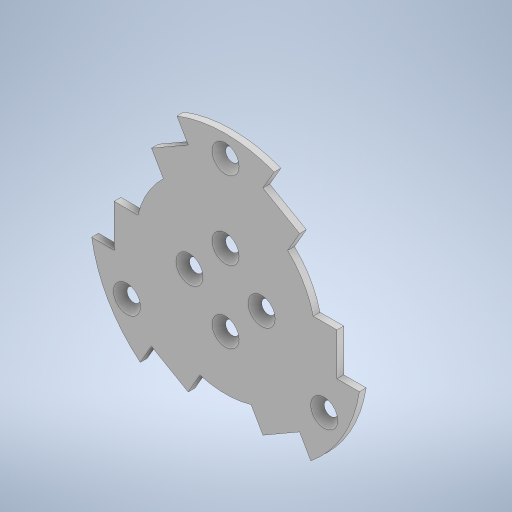
# Autodesk Inventor part: top_part_wheel
Saved by Autodesk Inventor 2023 (Build 270158000, 158)
## iProperties
Created: 2026-02-22
Part Number: top_part_wheel
Material: Типовые
Document SubType Name: Modeling
Designer: garin
Density: 1 g/cm^3
Appearance: По умолчанию
Author: garin
Autodesk Inventor part; units mm, degrees
ref_plane "YZ Plane" through (0, 0, 0) normal (1, 0, 0) x (0, 1, 0)
sketch "Эскиз1" plane through (0, 0, 0) normal (0, 0, 1) x (1, 0, 0)
  circle A0 centre (0, 0) radius 35
  circle A1 centre (0, 0) radius 20
  line L0 (0, 0) -> (34.5691, 5.4752) construction
  line L1 (0, 0) -> (35, 0) construction
  line L2 (0, 0) -> (34.5691, -5.4752) construction
  line L3 (34.5691, 5.4752) -> (29.6307, 4.693) construction
  line L4 (29.6307, 4.693) -> (19.4416, 4.693)
  line L5 (19.4416, 4.693) -> (34.6839, 4.693)
  line L6 (19.4416, -4.693) -> (34.6839, -4.693)
  line L7 (13.7851, 14.4904) -> (21.4063, 27.6907) construction
  line L8 (10.751, 28.0074) -> (5.6565, 19.1834) construction
  line L9 (5.6565, 19.1834) -> (13.2777, 32.3837) construction
  line L10 (-5.6565, 19.1834) -> (-13.2777, 32.3837) construction
  line L11 (-18.8796, 23.3144) -> (-13.7851, 14.4904) construction
  line L12 (-13.7851, 14.4904) -> (-21.4063, 27.6907) construction
  line L13 (-19.4416, 4.693) -> (-34.6839, 4.693) construction
  line L14 (-29.6307, -4.693) -> (-19.4416, -4.693) construction
  line L15 (-19.4416, -4.693) -> (-34.6839, -4.693) construction
  line L16 (-13.7851, -14.4904) -> (-21.4063, -27.6907) construction
  line L17 (-10.751, -28.0074) -> (-5.6565, -19.1834) construction
  line L18 (-5.6565, -19.1834) -> (-13.2777, -32.3837) construction
  line L19 (5.6565, -19.1834) -> (13.2777, -32.3837) construction
  line L20 (18.8796, -23.3144) -> (13.7851, -14.4904) construction
  line L21 (13.7851, -14.4904) -> (21.4063, -27.6907) construction
  line L22 (0, 0) -> (17.5, 30.3109) construction
  line L23 (0, 0) -> (-17.5, 30.3109) construction
  line L24 (0, 0) -> (-35, 0) construction
  line L25 (0, 0) -> (-17.5, -30.3109) construction
  line L26 (0, 0) -> (17.5, -30.3109) construction
  line L27 (34.6839, 4.693) -> (29.6839, 4.693) construction
  line L28 (29.6839, 4.693) -> (29.6839, -4.693)
  line L29 (29.6839, 4.693) -> (29.6839, 1.693)
  line L30 (29.6839, 1.693) -> (34.959, 1.693)
  line L31 (29.6839, -4.693) -> (29.6839, -1.693) construction
  line L32 (29.6839, -1.693) -> (34.959, -1.693)
  line L33 (13.7851, 14.4904) -> (21.4063, 27.6907)
  line L34 (10.751, 28.0074) -> (5.6565, 19.1834)
  line L35 (13.3758, 26.5536) -> (16.0133, 31.1219)
  line L36 (5.6565, 19.1834) -> (13.2777, 32.3837)
  line L37 (10.7777, 28.0536) -> (18.9063, 23.3605)
  line L38 (16.3082, 24.8605) -> (18.9457, 29.4289)
  line L39 (-5.6565, 19.1834) -> (-13.2777, 32.3837)
  line L40 (-18.8796, 23.3144) -> (-13.7851, 14.4904)
  line L41 (-16.3082, 24.8605) -> (-18.9457, 29.4289)
  line L42 (-13.7851, 14.4904) -> (-21.4063, 27.6907)
  line L43 (-18.9063, 23.3605) -> (-10.7777, 28.0536)
  line L44 (-13.3758, 26.5536) -> (-16.0133, 31.1219)
  line L45 (-19.4416, 4.693) -> (-34.6839, 4.693)
  line L46 (-29.6307, -4.693) -> (-19.4416, -4.693)
  line L47 (-29.6839, -1.693) -> (-34.959, -1.693)
  line L48 (-19.4416, -4.693) -> (-34.6839, -4.693)
  line L49 (-29.6839, -4.693) -> (-29.6839, 4.693)
  line L50 (-29.6839, 1.693) -> (-34.959, 1.693)
  line L51 (-13.7851, -14.4904) -> (-21.4063, -27.6907)
  line L52 (-10.751, -28.0074) -> (-5.6565, -19.1834)
  line L53 (-13.3758, -26.5536) -> (-16.0133, -31.1219)
  line L54 (-5.6565, -19.1834) -> (-13.2777, -32.3837)
  line L55 (-10.7777, -28.0536) -> (-18.9063, -23.3605)
  line L56 (-16.3082, -24.8605) -> (-18.9457, -29.4289)
  line L57 (5.6565, -19.1834) -> (13.2777, -32.3837)
  line L58 (18.8796, -23.3144) -> (13.7851, -14.4904)
  line L59 (16.3082, -24.8605) -> (18.9457, -29.4289)
  line L60 (13.7851, -14.4904) -> (21.4063, -27.6907)
  line L61 (18.9063, -23.3605) -> (10.7777, -28.0536)
  line L62 (13.3758, -26.5536) -> (16.0133, -31.1219)
  circle A2 centre (0, 0) radius 30.0525
  line L63 (21.4063, 27.6907) -> (19.9136, 25.1053) construction
  line L64 (18.9457, 29.4289) -> (17.4457, 26.8308) construction
  line L65 (17.4457, 26.8308) -> (21.2118, 27.8399)
  line L66 (0, 0) -> (21.2118, 27.8399) construction
  line L67 (21.2384, 23.9411) -> (21.2118, 27.8399)
  line L68 (24.7499, 20.2901) -> (25.3388, 24.1443)
  line L69 (21.4607, 23.742) -> (25.3388, 24.1443)
  line L70 (27.6414, 16.1308) -> (28.831, 19.8437)
  line L71 (24.938, 20.0584) -> (28.831, 19.8437)
  line L72 (29.8403, 11.5673) -> (31.6009, 15.046)
  line L73 (27.7906, 15.8723) -> (31.6009, 15.046)
  line L74 (31.2917, 6.714) -> (33.5791, 9.8714)
  line L75 (29.9469, 11.2885) -> (33.5791, 9.8714)
  line L76 (31.9591, 1.6925) -> (34.716, 4.4494)
  line L77 (31.3529, 6.4219) -> (34.716, 4.4494)
  circle A3 centre (0, 0) radius 32.0038
  line L78 (-14.5133, 28.5238) -> (-13.5042, 32.2899)
  line L79 (-10.1144, 30.3635) -> (-13.5042, 32.2899)
  line L80 (-9.8308, 30.4565) -> (-8.2401, 34.0162)
  line L81 (-5.1968, 31.5791) -> (-8.2401, 34.0162)
  line L82 (14.5138, 28.5236) -> (13.5047, 32.2897)
  line L83 (10.1149, 30.3634) -> (13.5047, 32.2897)
  line L84 (9.8313, 30.4564) -> (8.2407, 34.016)
  line L85 (5.1973, 31.579) -> (8.2407, 34.016)
  line L86 (4.9026, 31.6261) -> (2.7702, 34.8902)
  line L87 (0.1495, 32.0035) -> (2.7702, 34.8902)
  line L88 (-0.149, 32.0035) -> (-2.7697, 34.8902)
  line L89 (-4.9021, 31.6262) -> (-2.7697, 34.8902)
  line L90 (-31.959, 1.693) -> (-34.716, 4.45)
  line L91 (-31.3528, 6.4224) -> (-34.716, 4.45)
  line L92 (-31.2916, 6.7145) -> (-33.5789, 9.8719)
  line L93 (-29.9467, 11.289) -> (-33.5789, 9.8719)
  line L94 (-17.4453, 26.8311) -> (-21.2113, 27.8403)
  line L95 (-21.238, 23.9415) -> (-21.2113, 27.8403)
  line L96 (-21.4603, 23.7424) -> (-25.3384, 24.1447)
  line L97 (-24.7496, 20.2905) -> (-25.3384, 24.1447)
  line L98 (-24.9377, 20.0588) -> (-28.8307, 19.8442)
  line L99 (-27.6411, 16.1312) -> (-28.8307, 19.8442)
  line L100 (-27.7903, 15.8727) -> (-31.6007, 15.0465)
  line L101 (-29.8401, 11.5678) -> (-31.6007, 15.0465)
  line L102 (-17.4457, -26.8308) -> (-21.2118, -27.8399)
  line L103 (-21.2384, -23.9411) -> (-21.2118, -27.8399)
  line L104 (-21.4607, -23.742) -> (-25.3388, -24.1443)
  line L105 (-24.7499, -20.2901) -> (-25.3388, -24.1443)
  line L106 (-31.9591, -1.6925) -> (-34.716, -4.4494)
  line L107 (-31.3529, -6.4219) -> (-34.716, -4.4494)
  line L108 (-31.2917, -6.714) -> (-33.5791, -9.8714)
  line L109 (-29.9469, -11.2885) -> (-33.5791, -9.8714)
  line L110 (-29.8403, -11.5673) -> (-31.6009, -15.046)
  line L111 (-27.7906, -15.8723) -> (-31.6009, -15.046)
  line L112 (-27.6414, -16.1308) -> (-28.831, -19.8437)
  line L113 (-24.938, -20.0584) -> (-28.831, -19.8437)
  line L114 (14.5133, -28.5238) -> (13.5042, -32.2899)
  line L115 (10.1144, -30.3635) -> (13.5042, -32.2899)
  line L116 (9.8308, -30.4565) -> (8.2401, -34.0162)
  line L117 (5.1968, -31.5791) -> (8.2401, -34.0162)
  line L118 (-14.5138, -28.5236) -> (-13.5047, -32.2897)
  line L119 (-10.1149, -30.3634) -> (-13.5047, -32.2897)
  line L120 (-9.8313, -30.4564) -> (-8.2407, -34.016)
  line L121 (-5.1973, -31.579) -> (-8.2407, -34.016)
  line L122 (-4.9026, -31.6261) -> (-2.7702, -34.8902)
  line L123 (-0.1495, -32.0035) -> (-2.7702, -34.8902)
  line L124 (0.149, -32.0035) -> (2.7697, -34.8902)
  line L125 (4.9021, -31.6262) -> (2.7697, -34.8902)
  line L126 (31.959, -1.693) -> (34.716, -4.45)
  line L127 (31.3528, -6.4224) -> (34.716, -4.45)
  line L128 (31.2916, -6.7145) -> (33.5789, -9.8719)
  line L129 (29.9467, -11.289) -> (33.5789, -9.8719)
  line L130 (17.4453, -26.8311) -> (21.2113, -27.8403)
  line L131 (21.238, -23.9415) -> (21.2113, -27.8403)
  line L132 (21.4603, -23.7424) -> (25.3384, -24.1447)
  line L133 (24.7496, -20.2905) -> (25.3384, -24.1447)
  line L134 (24.9377, -20.0588) -> (28.8307, -19.8442)
  line L135 (27.6411, -16.1312) -> (28.8307, -19.8442)
  line L136 (27.7903, -15.8727) -> (31.6007, -15.0465)
  line L137 (29.8401, -11.5678) -> (31.6007, -15.0465)
  circle A4 centre (0, 0) radius 11 construction
  line L138 (0, 0) -> (0, 8) construction
  circle A5 centre (0, 8) radius 1.5
  circle A6 centre (0, -8) radius 1.5
  line L139 (0, 0) -> (8, 0) construction
  circle A7 centre (8, 0) radius 1.5
  circle A8 centre (-8, 0) radius 1.5
  circle A9 centre (0, 0) radius 12.5
  line L140 (-10.751, -28.0074) -> (-9.251, -25.4093)
  circle A10 centre (0, 0) radius 27.041
  line L141 (24.7024, 4.693) -> (24.7024, -4.693)
  line L142 (8.2869, 23.7395) -> (16.4155, 19.0464)
  line L143 (-16.4155, 19.0464) -> (-8.2869, 23.7395)
  line L144 (-24.7024, -4.693) -> (-24.7024, 4.693)
  line L145 (-8.2869, -23.7395) -> (-16.4155, -19.0464)
  line L146 (16.4155, -19.0464) -> (8.2869, -23.7395)
  line L147 (-13.7851, -14.4904) -> (-18.9063, -23.3605)
  line L148 (-19.4416, -4.693) -> (-29.6839, -4.693)
  arc A11 (-24.5628, -4.693) -> (-16.3457, -18.9255) centre (-3.3046, -1.9079) ccw
  circle A12 centre (-21.872, -12.6278) radius 1.5
  circle A13 centre (21.872, -12.6278) radius 1.5
  circle A14 centre (0, 25.2557) radius 1.5
  line L149 (-16.3457, -18.9255) -> (-17.3796, -20.7163)
  line L150 (-16.4155, -19.0464) -> (-18.9063, -23.3605)
  line L151 (-24.7024, -4.693) -> (-29.6839, -4.693)
  line L152 (-24.7024, -4.693) -> (-29.6839, -4.693)
  arc A15 (-29.6839, -4.693) -> (-18.9063, -23.3605) centre (0.0018, 0.001) ccw
  arc A16 (-19.4416, -4.693) -> (-13.7851, -14.4904) centre (0, 0) ccw
  line L153 (-29.6839, -4.693) -> (-19.4416, -4.693)
  line L154 (18.8796, -23.3144) -> (13.7851, -14.4904)
  line L155 (19.4416, -4.693) -> (29.6839, -4.693)
  arc A17 (18.9063, -23.3605) -> (29.6839, -4.693) centre (-0.0018, 0.001) ccw
  line L156 (10.751, 28.0074) -> (5.6565, 19.1834)
  line L157 (-5.6565, 19.1834) -> (-10.7777, 28.0536)
  arc A18 (10.7777, 28.0536) -> (-10.7777, 28.0536) centre (0, -0.0021) ccw
  point P0 (18.9062, 23.3604)
  point P1 (18.9055, 23.3609)
  point P2 (10.7784, 28.0531)
  point P3 (10.7776, 28.0534)
  point P4 (-10.7776, 28.0534)
  point P5 (-10.7784, 28.0531)
  point P6 (-18.9055, 23.3609)
  point P7 (-18.9062, 23.3604)
  point P8 (-29.6838, 4.693)
  point P9 (-29.6839, 4.6922)
  point P10 (-29.6839, -4.6922)
  point P11 (-29.6838, -4.693)
  point P12 (-18.9062, -23.3604)
  point P13 (-18.9055, -23.3609)
  point P14 (-10.7784, -28.0531)
  point P15 (-10.7776, -28.0534)
  point P16 (10.7776, -28.0534)
  point P17 (10.7784, -28.0531)
  point P18 (18.9055, -23.3609)
  point P19 (18.9062, -23.3604)
  point P20 (29.6838, -4.693)
  point P21 (29.6839, -4.6922)
  point P22 (29.6839, 4.6922)
  point P23 (29.6838, 4.693)
  point P24 (17.3796, 20.7163)
  point P25 (9.251, 25.4093)
  point P26 (-9.251, 25.4093)
  point P27 (-17.3796, 20.7163)
  point P28 (-26.6307, 4.693)
  point P29 (-26.6307, -4.693)
  point P30 (-17.3796, -20.7163)
  point P31 (9.251, -25.4093)
  point P32 (17.3796, -20.7163)
  point P33 (26.6307, -4.693)
  point P34 (26.6307, 4.693)
  point P35 (21.4063, -27.6907)
  point P36 (24.5628, -4.693)
  point P37 (26.6307, -4.693)
  point P38 (13.2777, 32.3837)
  point P39 (-8.2171, 23.6185)
  point P40 (-9.251, 25.4093)
  dimension "d11" = 40
  dimension "d21" = 60.105
  dimension "d10" = 70
  dimension "d12" = 9
  dimension "d13" = 5
  dimension "d14" = 360
  dimension "d15" = 360
  dimension "d16" = 5
  dimension "d17" = 90
  dimension "d18" = 3
  dimension "d19" = 3
  dimension "d20" = 360
  dimension "d22" = 3
  dimension "d23" = 45
  dimension "d24" = 45.392
  dimension "d25" = 360
  dimension "d26" = 22
  dimension "d27" = 8
  dimension "d28" = 3
  dimension "d29" = 8
  dimension "d30" = 3
  dimension "d31" = 25
  dimension "d37" = 3
  dimension "d40" = 360
  dimension "d42" = 3
  dimension "d45" = 360
  dimension "d49" = 360
  constraints: 316 end point, 49 point on line, 18 point on circle, 16 centre point, 9 coincident, 6 symmetric about line, 4 perpendicular, 3 horizontal, 2 collinear, 2 midpoint, 1 equal length, 1 vertical, 452 other
  measures "d10" diameter of A0
  measures "d12" angle of L1 L0
  measures "d13" distance of L0.end L4.start
  measures "d16" distance of L5.end L28.start
  measures "d17" angle of L28 L27
  measures "d18" distance of L28.start L29.end
  measures "d19" distance of L31.start L31.end
  measures "d22" distance of L38.end L65.start
  measures "d23" angle of L65 L64
  measures "d26" diameter of A4
  measures "d27" distance of L139.start L138.end
  measures "d28" diameter of A5
  measures "d29" distance of L139.start L139.end
  measures "d30" diameter of A7
  measures "d31" diameter of A9
  measures "d37" distance of L17.start L140.end
  measures "d42" diameter of A12
ref_plane "РабПлоскость1" through (-29.6838, -23.3604, 11) normal (0, 0, 1) x (1, 0, 0)
ref_plane "РабПлоскость2" through (-34.716, -34.8902, 12) normal (0, 0, 1) x (1, 0, 0)
extrude "Выдавливание1" add sketch "Эскиз1" along normal blind 1.5 from surface at 12 contours A2 L60 L58 A10 L6 | A10 L58 A1 L6 | L6 A1 L4 L141 | L33 A1 L34 L142 | A10 L39 A2 L36 L34 | L34 A1 L39 A10 | A1 | L146 L57 A1 L58 | L39 A1 L40 L143 | L145 L51 A1 L52 | A10 L46 A11 A12 L51 | L51 A2 L48 L46 A10 | L45 A1 L46 L144 | L51 A11 A12 L46 A1 | A9
chamfer "Фаска1" distance 1.5 angle 45 4 edges at (-9.5, 0, 13.5) (-1.5, -8, 13.5) (6.5, 0, 13.5) (-1.5, 8, 13.5)
sketch "Эскиз2" plane through (8.2869, -23.7395, 12) normal (0.5, -0.8660254, 0) x (0.8660254, 0.5, 0)
  point P0 (4.693, -12)
chamfer "Фаска2" distance 1.5 angle 45 3 edges at (20.372, -12.6278, 13.5) (-23.372, -12.6278, 13.5) (-1.5, 25.2557, 13.5)
